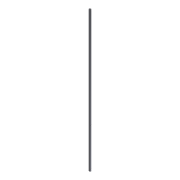
# Autodesk Inventor part: JointC1
Saved by Autodesk Inventor 2011 SP1 (Build 150282100, 282)
## iProperties
Created: 2012-10-16
Part Number: JointC1
Document SubType Name: Modeling
Designer: arihon
Density: 1 g/cm^3
Author: arihon
Autodesk Inventor part; units mm, degrees
ref_plane "YZ Plane" through (0, 0, 0) normal (1, 0, 0) x (0, 1, 0)
ref_plane "XZ Plane" through (0, 0, 0) normal (0, 1, 0) x (-1, 0, 0)
ref_plane "XY Plane" through (0, 0, 0) normal (0, 0, 1) x (1, 0, 0)
sketch "スケッチ1" plane through (0, 0, 0) normal (0, 0, 1) x (1, 0, 0)
  circle A0 centre (0, 0) radius 5
  circle A1 centre (0, 0) radius 4.5
  dimension "d0" = 10
  dimension "d1" = 9
  constraints: 2 centre point, 2 coincident
  measures "d0" diameter of A0
  measures "d1" diameter of A1
extrude "押し出し1" add sketch "スケッチ1" along normal blind 700
sketch "スケッチ2" plane through (0, 0, 0) normal (0, 0, -1) x (-1, 0, 0)
  circle A0 centre (0, 0) radius 5 projected
  line L0 (-4.9, 0.995) -> (-4.9, -0.995)
  dimension "d4" = 0.1
  constraints: 2 end point, 2 point on circle, 1 vertical
  measures "d4" distance edge to line of A0 L0
extrude "押し出し2" cut sketch "スケッチ2" against normal through all contours L0 A0 picked at (-4.9296, 0.1112)
sketch "スケッチ3" plane through (4.9, -0.995, 700) normal (1, 0, 0) x (0, 0, -1)
  line L0 (700, 1.99) -> (700, 0) projected
  point P0 (700, 0.995)
  point P1 (500, 0.995)
  point P2 (0, 0)
  point P3 (5, 0.995)
  point P4 (690, 0.995)
  dimension "d7" = 200
  dimension "d15" = 5
  dimension "d16" = 10
  measures "d7" distance from line of L0 point (500, 0.995)
  measures "d15" horizontal distance of point (0, 0) point (5, 0.995)
  measures "d16" distance of point (700, 0.995) point (690, 0.995)
hole "Hole1" at (4.9, 0, 200) at (4.9, 0, 695) at (4.9, 0, 10) direction (-1, 0, 0) diameter 3 end through all
